Autodesk Inventor part; units mm, degrees
(part 2 of 6)
  arc A582 (128.3559, 101.1967) -> (128.4338, 100.8049) centre (148.5, 105) ccw
  arc A583 (128.7164, 99.628) -> (128.8248, 99.2435) centre (148.5, 105) ccw
  arc A584 (129.1989, 98.0923) -> (129.3371, 97.7175) centre (148.5, 105) ccw
  arc A585 (129.8003, 96.5993) -> (129.9676, 96.2365) centre (148.5, 105) ccw
  arc A586 (130.5171, 95.158) -> (130.7123, 94.8095) centre (148.5, 105) ccw
  arc A587 (131.3447, 93.7774) -> (131.5666, 93.4453) centre (148.5, 105) ccw
  arc A588 (132.2781, 92.466) -> (132.5254, 92.1523) centre (148.5, 105) ccw
  arc A589 (133.3115, 91.2319) -> (133.5827, 90.9386) centre (148.5, 105) ccw
  arc A590 (134.4386, 90.0827) -> (134.7319, 89.8115) centre (148.5, 105) ccw
  arc A591 (135.6523, 89.0254) -> (135.966, 88.7781) centre (148.5, 105) ccw
  arc A592 (136.9453, 88.0666) -> (137.2774, 87.8447) centre (148.5, 105) ccw
  arc A593 (138.3095, 87.2123) -> (138.658, 87.0171) centre (148.5, 105) ccw
  arc A594 (139.7365, 86.4676) -> (140.0993, 86.3003) centre (148.5, 105) ccw
  arc A595 (141.2175, 85.8371) -> (141.5923, 85.6989) centre (148.5, 105) ccw
  arc A596 (142.7435, 85.3248) -> (143.128, 85.2164) centre (148.5, 105) ccw
  arc A597 (144.3049, 84.9338) -> (144.6967, 84.8559) centre (148.5, 105) ccw
  arc A598 (145.8922, 84.6665) -> (146.2889, 84.6196) centre (148.5, 105) ccw
  arc A599 (147.4956, 84.5246) -> (147.8948, 84.5089) centre (148.5, 105) ccw
  arc A600 (149.1052, 84.5089) -> (149.5044, 84.5246) centre (148.5, 105) ccw
  arc A601 (150.7111, 84.6196) -> (151.1078, 84.6665) centre (148.5, 105) ccw
  arc A602 (152.3033, 84.8559) -> (152.6951, 84.9338) centre (148.5, 105) ccw
  arc A603 (153.872, 85.2164) -> (154.2565, 85.3248) centre (148.5, 105) ccw
  arc A604 (155.4077, 85.6989) -> (155.7825, 85.8371) centre (148.5, 105) ccw
  arc A605 (156.9007, 86.3003) -> (157.2635, 86.4676) centre (148.5, 105) ccw
  arc A606 (158.342, 87.0171) -> (158.6905, 87.2123) centre (148.5, 105) ccw
  arc A607 (159.7226, 87.8447) -> (160.0547, 88.0666) centre (148.5, 105) ccw
  arc A608 (161.034, 88.7781) -> (161.3477, 89.0254) centre (148.5, 105) ccw
  arc A609 (162.2681, 89.8115) -> (162.5614, 90.0827) centre (148.5, 105) ccw
  arc A610 (163.4173, 90.9386) -> (163.6885, 91.2319) centre (148.5, 105) ccw
  arc A611 (164.4746, 92.1523) -> (164.7219, 92.466) centre (148.5, 105) ccw
  arc A612 (165.4334, 93.4453) -> (165.6553, 93.7774) centre (148.5, 105) ccw
  arc A613 (166.2877, 94.8095) -> (166.4829, 95.158) centre (148.5, 105) ccw
  arc A614 (167.0324, 96.2365) -> (167.1997, 96.5993) centre (148.5, 105) ccw
  arc A615 (167.6629, 97.7175) -> (167.8011, 98.0923) centre (148.5, 105) ccw
  arc A616 (168.1752, 99.2435) -> (168.2836, 99.628) centre (148.5, 105) ccw
  arc A617 (168.5662, 100.8049) -> (168.6441, 101.1967) centre (148.5, 105) ccw
  arc A618 (168.8335, 102.3922) -> (168.8804, 102.7889) centre (148.5, 105) ccw
  arc A619 (168.9754, 103.9956) -> (168.9911, 104.3948) centre (148.5, 105) ccw
  arc A620 (168.9911, 105.6052) -> (168.9754, 106.0044) centre (148.5, 105) ccw
  arc A621 (168.8804, 107.2111) -> (168.8335, 107.6078) centre (148.5, 105) ccw
  arc A622 (168.6441, 108.8033) -> (168.5662, 109.1951) centre (148.5, 105) ccw
  arc A623 (168.2836, 110.372) -> (168.1752, 110.7565) centre (148.5, 105) ccw
  arc A624 (167.8011, 111.9077) -> (167.6629, 112.2825) centre (148.5, 105) ccw
  arc A625 (167.1997, 113.4007) -> (167.0324, 113.7635) centre (148.5, 105) ccw
  arc A626 (166.4829, 114.842) -> (166.2877, 115.1905) centre (148.5, 105) ccw
  arc A627 (165.6553, 116.2226) -> (165.4334, 116.5547) centre (148.5, 105) ccw
  arc A628 (164.7219, 117.534) -> (164.4746, 117.8477) centre (148.5, 105) ccw
  arc A629 (163.6885, 118.7681) -> (163.4173, 119.0614) centre (148.5, 105) ccw
  arc A630 (162.5614, 119.9173) -> (162.2681, 120.1885) centre (148.5, 105) ccw
  arc A631 (161.3477, 120.9746) -> (161.034, 121.2219) centre (148.5, 105) ccw
  arc A632 (160.0547, 121.9334) -> (159.7226, 122.1553) centre (148.5, 105) ccw
  arc A633 (158.6905, 122.7877) -> (158.342, 122.9829) centre (148.5, 105) ccw
  arc A634 (157.2635, 123.5324) -> (156.9007, 123.6997) centre (148.5, 105) ccw
  arc A635 (155.7825, 124.1629) -> (155.4077, 124.3011) centre (148.5, 105) ccw
  arc A636 (154.2565, 124.6752) -> (153.872, 124.7836) centre (148.5, 105) ccw
  arc A637 (152.6951, 125.0662) -> (152.3033, 125.1441) centre (148.5, 105) ccw
  arc A638 (151.1078, 125.3335) -> (150.7111, 125.3804) centre (148.5, 105) ccw
  arc A639 (149.5044, 125.4754) -> (149.1052, 125.4911) centre (148.5, 105) ccw
  line L0 (126, 105) -> (171, 105)
  line L1 (148.5, 82.5) -> (148.5, 127.5)
  line L2 (189, 125.5) -> (259, 125.5)
  line L3 (189, 117.5) -> (259, 117.5)
  line L4 (189, 109.5) -> (259, 109.5)
  line L5 (189, 101.5) -> (259, 101.5)
  line L6 (189, 93.5) -> (259, 93.5)
  line L7 (189, 85.5) -> (259, 85.5)
  line L8 (189, 77.5) -> (259, 77.5)
  line L9 (189, 69.5) -> (259, 69.5)
  line L10 (189, 61.5) -> (259, 61.5)
  line L11 (189, 53.5) -> (259, 53.5)
  line L12 (189, 45.5) -> (259, 45.5)
  line L13 (189, 37.5) -> (259, 37.5)
  line L14 (189, 29.5) -> (259, 29.5)
  line L15 (189, 125.5) -> (189, 29.5)
  line L16 (259, 125.5) -> (259, 29.5)
  line L17 (224, 117.5) -> (224, 29.5)
  arc A640 (149.1982, 109.7586) -> (149.1615, 109.6213) centre (149.7545, 109.5365) ccw
  arc A641 (149.402, 110.1264) -> (149.1982, 109.7586) centre (150.7515, 109.1382) ccw
  arc A642 (150.0725, 110.7903) -> (149.402, 110.1264) centre (151.8157, 108.3591) ccw
  arc A643 (146.2672, 109.2599) -> (146.3182, 109.1272) centre (146.8478, 109.4071) ccw
  arc A644 (146.2159, 109.6791) -> (146.2672, 109.2599) centre (147.8885, 109.671) ccw
  arc A645 (146.3688, 110.6087) -> (146.2159, 109.6791) centre (149.2074, 109.6645) ccw
  arc A646 (144.1897, 107.1339) -> (144.309, 107.0566) centre (144.5729, 107.5943) ccw
  arc A647 (143.9018, 107.4429) -> (144.1897, 107.1339) centre (145.2598, 108.4195) ccw
  arc A648 (143.4791, 108.2848) -> (143.9018, 107.4429) centre (146.3305, 109.1895) ccw
  arc A649 (143.7586, 104.1928) -> (143.9006, 104.2004) centre (143.7981, 104.7905) ccw
  arc A650 (143.3441, 104.2736) -> (143.7586, 104.1928) centre (143.8687, 105.8619) ccw
  arc A651 (142.5072, 104.7063) -> (143.3441, 104.2736) centre (144.2823, 107.1142) ccw
  arc A652 (145.1386, 101.5601) -> (145.249, 101.6496) centre (144.8192, 102.0668) ccw
  arc A653 (144.7558, 101.3818) -> (145.1386, 101.5601) centre (144.2466, 102.9751) ccw
  arc A654 (143.8244, 101.2399) -> (144.7558, 101.3818) centre (143.8452, 104.2313) ccw
  arc A655 (147.8018, 100.2415) -> (147.8385, 100.3788) centre (147.2456, 100.4636) ccw
  arc A656 (147.5969, 99.8722) -> (147.8018, 100.2415) centre (146.2485, 100.8619) ccw
  arc A657 (146.9268, 99.2099) -> (147.5969, 99.8722) centre (145.1853, 101.6423) ccw
  arc A658 (150.7315, 100.7396) -> (150.6805, 100.8723) centre (150.1509, 100.5924) ccw
  arc A659 (150.7828, 100.3204) -> (150.7315, 100.7396) centre (149.1102, 100.3285) ccw
  arc A660 (150.6299, 99.3908) -> (150.7828, 100.3204) centre (147.7913, 100.335) ccw
  arc A661 (152.8095, 102.8649) -> (152.6903, 102.9423) centre (152.4263, 102.4046) ccw
  arc A662 (153.0974, 102.5559) -> (152.8095, 102.8649) centre (151.7394, 101.5794) ccw
  arc A663 (153.5202, 101.714) -> (153.0974, 102.5559) centre (150.6687, 100.8093) ccw
  arc A664 (153.2414, 105.8058) -> (153.0995, 105.7982) centre (153.202, 105.2081) ccw
  arc A665 (153.656, 105.725) -> (153.2414, 105.8058) centre (153.1314, 104.1367) ccw
  arc A666 (154.4929, 105.2923) -> (153.656, 105.725) centre (152.7177, 102.8844) ccw
  arc A667 (151.8623, 108.4388) -> (151.7519, 108.3493) centre (152.1817, 107.9321) ccw
  arc A668 (152.2451, 108.6171) -> (151.8623, 108.4388) centre (152.7543, 107.0239) ccw
  arc A669 (153.1765, 108.759) -> (152.2451, 108.6171) centre (153.1557, 105.7676) ccw
  arc A670 (147.8392, 109.6213) -> (147.8025, 109.7587) centre (147.2462, 109.5365) ccw
  arc A671 (147.8025, 109.7587) -> (147.5976, 110.128) centre (146.2492, 109.1383) ccw
  arc A672 (147.5976, 110.128) -> (146.9275, 110.7903) centre (145.186, 108.3579) ccw
  arc A673 (145.2491, 108.3503) -> (145.1386, 108.4399) centre (144.8192, 107.9332) ccw
  arc A674 (145.1386, 108.4399) -> (144.7558, 108.6182) centre (144.2466, 107.0249) ccw
  arc A675 (144.7558, 108.6182) -> (143.8244, 108.7601) centre (143.8452, 105.7687) ccw
  arc A676 (143.9007, 105.7996) -> (143.7586, 105.8072) centre (143.7981, 105.2095) ccw
  arc A677 (143.7586, 105.8072) -> (143.3441, 105.7264) centre (143.8687, 104.1381) ccw
  arc A678 (143.3441, 105.7264) -> (142.5072, 105.2937) centre (144.2823, 102.8858) ccw
  arc A679 (144.309, 102.9435) -> (144.1897, 102.8661) centre (144.5729, 102.4057) ccw
  arc A680 (144.1897, 102.8661) -> (143.9018, 102.5571) centre (145.2598, 101.5805) ccw
  arc A681 (143.9018, 102.5571) -> (143.4791, 101.7152) centre (146.3305, 100.8105) ccw
  arc A682 (146.3189, 100.8726) -> (146.2679, 100.7399) centre (146.8485, 100.5927) ccw
  arc A683 (146.2679, 100.7399) -> (146.2166, 100.3207) centre (147.8892, 100.3288) ccw
  arc A684 (146.2166, 100.3207) -> (146.3695, 99.391) centre (149.2081, 100.3352) ccw
  arc A685 (149.1608, 100.3787) -> (149.1975, 100.2413) centre (149.7538, 100.4635) ccw
  arc A686 (149.1975, 100.2413) -> (149.4024, 99.872) centre (150.7508, 100.8617) ccw
  arc A687 (149.4024, 99.872) -> (150.0725, 99.2097) centre (151.814, 101.6421) ccw
  arc A688 (151.7509, 101.6497) -> (151.8614, 101.5601) centre (152.1808, 102.0668) ccw
  arc A689 (151.8614, 101.5601) -> (152.2442, 101.3818) centre (152.7534, 102.9751) ccw
  arc A690 (152.2442, 101.3818) -> (153.1756, 101.2399) centre (153.1548, 104.2313) ccw
  arc A691 (153.0993, 104.2004) -> (153.2414, 104.1928) centre (153.2019, 104.7905) ccw
  arc A692 (153.2414, 104.1928) -> (153.6559, 104.2736) centre (153.1313, 105.8619) ccw
  arc A693 (153.6559, 104.2736) -> (154.4928, 104.7063) centre (152.7177, 107.1142) ccw
  arc A694 (152.691, 107.0565) -> (152.8103, 107.1339) centre (152.4271, 107.5943) ccw
  arc A695 (152.8103, 107.1339) -> (153.0982, 107.4429) centre (151.7402, 108.4195) ccw
  arc A696 (153.0982, 107.4429) -> (153.5209, 108.2848) centre (150.6695, 109.1895) ccw
  arc A697 (150.6818, 109.1272) -> (150.7328, 109.2599) centre (150.1522, 109.4071) ccw
  arc A698 (150.7328, 109.2599) -> (150.7841, 109.6791) centre (149.1115, 109.671) ccw
  arc A699 (150.7841, 109.6791) -> (150.6312, 110.6087) centre (147.7926, 109.6645) ccw
  arc A700 (149.0314, 108.7125) -> (147.9691, 108.7126) centre (148.5, 105) ccw
  arc A701 (146.7471, 108.3155) -> (145.8883, 107.6915) centre (148.5, 105) ccw
  arc A702 (145.1331, 106.652) -> (144.8051, 105.6424) centre (148.5, 105) ccw
  arc A703 (144.8051, 104.3575) -> (145.1332, 103.3479) centre (148.5, 105) ccw
  arc A704 (145.8884, 102.3084) -> (146.7478, 101.6841) centre (148.5, 105) ccw
  arc A705 (147.9686, 101.2875) -> (149.0308, 101.2874) centre (148.5, 105) ccw
  arc A706 (150.2516, 101.6838) -> (151.1117, 102.3085) centre (148.5, 105) ccw
  arc A707 (151.8663, 103.3467) -> (152.1949, 104.3576) centre (148.5, 105) ccw
  arc A708 (152.1951, 105.6411) -> (151.8668, 106.6521) centre (148.5, 105) ccw
  arc A709 (151.1126, 107.6906) -> (150.2528, 108.3155) centre (148.5, 105) ccw
  arc A710 (146.9275, 110.7903) -> (146.3688, 110.6087) centre (148.5, 105) ccw
  arc A711 (143.8244, 108.7601) -> (143.4791, 108.2848) centre (148.5, 105) ccw
  arc A712 (142.5072, 105.2937) -> (142.5072, 104.7063) centre (148.5, 105) ccw
  arc A713 (143.4791, 101.7152) -> (143.8244, 101.2399) centre (148.5, 105) ccw
  arc A714 (146.3695, 99.391) -> (146.9268, 99.2099) centre (148.5, 105) ccw
  arc A715 (150.0725, 99.2097) -> (150.6299, 99.3908) centre (148.5, 105) ccw
  arc A716 (153.1756, 101.2399) -> (153.5202, 101.714) centre (148.5, 105) ccw
  arc A717 (154.4928, 104.7063) -> (154.4929, 105.2923) centre (148.5, 105) ccw
  arc A718 (153.5209, 108.2848) -> (153.1765, 108.759) centre (148.5, 105) ccw
  arc A719 (150.6312, 110.6087) -> (150.0725, 110.7903) centre (148.5, 105) ccw
  line L18 (149.0314, 108.7125) -> (149.1615, 109.6213)
  line L19 (146.7471, 108.3155) -> (146.3182, 109.1272)
  line L20 (145.1331, 106.652) -> (144.309, 107.0566)
  line L21 (144.8051, 104.3575) -> (143.9006, 104.2004)
  line L22 (145.8884, 102.3084) -> (145.249, 101.6496)
  line L23 (147.9686, 101.2875) -> (147.8385, 100.3788)
  line L24 (150.2516, 101.6838) -> (150.6805, 100.8723)
  line L25 (151.8663, 103.3467) -> (152.6903, 102.9423)
  line L26 (152.1951, 105.6411) -> (153.0995, 105.7982)
  line L27 (151.1126, 107.6906) -> (151.7519, 108.3493)
  line L28 (147.9691, 108.7126) -> (147.8392, 109.6213)
  line L29 (145.8883, 107.6915) -> (145.2491, 108.3503)
  line L30 (144.8051, 105.6424) -> (143.9007, 105.7996)
  line L31 (145.1332, 103.3479) -> (144.309, 102.9435)
  line L32 (146.7478, 101.6841) -> (146.3189, 100.8726)
  line L33 (149.0308, 101.2874) -> (149.1608, 100.3787)
  line L34 (151.1117, 102.3085) -> (151.7509, 101.6497)
  line L35 (152.1949, 104.3576) -> (153.0993, 104.2004)
  line L36 (151.8668, 106.6521) -> (152.691, 107.0565)
  line L37 (150.2528, 108.3155) -> (150.6818, 109.1272)
  line L38 (140.5, 105) -> (156.5, 105)
  line L39 (148.5, 97) -> (148.5, 113)
  line L40 (174.5, 111) -> (244.5, 111)
  line L41 (174.5, 103) -> (244.5, 103)
  line L42 (174.5, 95) -> (244.5, 95)
  line L43 (174.5, 87) -> (244.5, 87)
  line L44 (174.5, 79) -> (244.5, 79)
  line L45 (174.5, 71) -> (244.5, 71)
  line L46 (174.5, 63) -> (244.5, 63)
  line L47 (174.5, 55) -> (244.5, 55)
  line L48 (174.5, 47) -> (244.5, 47)
  line L49 (174.5, 39) -> (244.5, 39)
  line L50 (174.5, 31) -> (244.5, 31)
  line L51 (174.5, 23) -> (244.5, 23)
  line L52 (174.5, 15) -> (244.5, 15)
  line L53 (174.5, 111) -> (174.5, 15)
  line L54 (244.5, 111) -> (244.5, 15)
  line L55 (209.5, 103) -> (209.5, 15)
  point P0 (0, 0)
  point P1 (195, 119.5)
  point P2 (197.5, 111.5)
  point P3 (197.5, 103.5)
  point P4 (195, 95.5)
  point P5 (197.5, 87.5)
  point P6 (192.5, 79.5)
  point P7 (195, 71.5)
  point P8 (195, 63.5)
  point P9 (195, 55.5)
  point P10 (197.5, 47.5)
  point P11 (197.5, 39.5)
  point P12 (195, 31.5)
  point P13 (225, 111.5)
  point P14 (240, 103.5)
  point P15 (238.75, 95.5)
  point P16 (237.5, 87.5)
  point P17 (240, 79.5)
  point P18 (233.75, 71.5)
  point P19 (240, 63.5)
  point P20 (236.25, 55.5)
  point P21 (235, 47.5)
  point P22 (242.5, 39.5)
  point P23 (242.5, 31.5)
  point P24 (149.5, 141)
  point P25 (149.5, 135)
  point P26 (165.6875, 141)
  point P27 (167.8125, 135)
  point P28 (180.5, 105)
  point P29 (183, 97)
  point P30 (183, 89)
  point P31 (180.5, 81)
  point P32 (183, 73)
  point P33 (178, 65)
  point P34 (180.5, 57)
  point P35 (180.5, 49)
  point P36 (180.5, 41)
  point P37 (183, 33)
  point P38 (183, 25)
  point P39 (180.5, 17)
  point P40 (210.5, 97)
  point P41 (225.5, 89)
  point P42 (226.75, 81)
  point P43 (223, 73)
  point P44 (225.5, 65)
  point P45 (220.5, 57)
  point P46 (225.5, 49)
  point P47 (224.25, 41)
  point P48 (220.5, 33)
  point P49 (228, 25)
  point P50 (228, 17)
  point P51 (149.5, 126.5)
  point P52 (149.5, 120.5)
  point P53 (167.8125, 126.5)
  point P54 (168.875, 120.5)
  constraints: 1120 point on circle, 560 centre point, 534 equal radius, 410 tangent, 104 end point, 84 horizontal, 26 parallel, 9 concentric, 4 midpoint, 4 perpendicular, 2 horizontal alignment, 2 vertical alignment, 586 other
extrude "押し出し1" add sketch "スケッチ1" along normal blind 3 contours A1 A2 A639 A479 A478 A477 A559 A237 A238 A239 A638 A476 A475 A474 A558 A234 A235 A236 A637 A473 A472 A471 A557 A231 A232 A233 A636 A470 A469 A468 A556 A228 A229 A230 A635 A467 A466 A465 A555 A225 A226 A227 A634 A464 A463 A462 A554 A222 A223 A224 A633 A461 A460 A459 A553 A219 A220 A221 A632 A458 A457 A456 A552 A216 A217 A218 A631 A455 A454 A453 A551 A213 A214 A215 A630 A452 A451 A450 A550 A210 A211 A212 A629 A449 A448 A447 A549 A207 A208 A209 A628 A446 A445 A444 A548 A204 A205 A206 A627 A443 A442 A441 A547 A201 A202 A203 A626 A440 A439 A438 A546 A198 A199 A200 A625 A437 A436 A435 A545 A195 A196 A197 A624 A434 A433 A432 A544 A192 A193 A194 A623 A431 A430 A429 A543 A189 A190 A191 A622 A428 A427 A426 A542 A186 A187 A188 A621 A425 A424 A423 A541 A183 A184 A185 A620 A422 A421 A420 A540 L0 A717 A666 A665 A664 L26 A708 L36 A694 A695 A696 A718 A669 A668 A667 L27 A709 L37 A697 A698 A699 A719 A642 A641 A640 L18 A700 L1 A480 A0 | L1 A700 L28 A670 A671 A672 A710 A645 A644 A643 L19 A701 L29 A673 A674 A675 A711 A648 A647 A646 L20 A702 L30 A676 A677 A678 A712 L0 A500 A60 A61 A62 A579 A299 A298 A297 A499 A57 A58 A59 A578 A296 A295 A294 A498 A54 A55 A56 A577 A293 A292 A291 A497 A51 A52 A53 A576 A290 A289 A288 A496 A48 A49 A50 A575 A287 A286 A285 A495 A45 A46 A47 A574 A284 A283 A282 A494 A42 A43 A44 A573 A281 A280 A279 A493 A39 A40 A41 A572 A278 A277 A276 A492 A36 A37 A38 A571 A275 A274 A273 A491 A33 A34 A35 A570 A272 A271 A270 A490 A30 A31 A32 A569 A269 A268 A267 A489 A27 A28 A29 A568 A266 A265 A264 A488 A24 A25 A26 A567 A263 A262 A261 A487 A21 A22 A23 A566 A260 A259 A258 A486 A18 A19 A20 A565 A257 A256 A255 A485 A15 A16 A17 A564 A254 A253 A252 A484 A12 A13 A14 A563 A251 A250 A249 A483 A9 A10 A11 A562 A248 A247 A246 A482 A6 A7 A8 A561 A245 A244 A243 A481 A3 A4 A5 A560 A242 A241 A240 A480 | A700 L18 A640 A641 A642 A719 A699 A698 A697 L37 A709 L27 A667 A668 A669 A718 A696 A695 A694 L36 A708 L26 A664 A665 A666 A717 L0 L1 | L1 L0 A712 A678 A677 A676 L30 A702 L20 A646 A647 A648 A711 A675 A674 A673 L29 A701 L19 A643 A644 A645 A710 A672 A671 A670 L28 A700 | L1 A705 L23 A655 A656 A657 A714 A684 A683 A682 L32 A704 L22 A652 A653 A654 A713 A681 A680 A679 L31 A703 L21 A649 A650 A651 A712 L0 | L0 A717 A693 A692 A691 L35 A707 L25 A661 A662 A663 A716 A690 A689 A688 L34 A706 L24 A658 A659 A660 A715 A687 A686 A685 L33 A705 L1 | A712 A651 A650 A649 L21 A703 L31 A679 A680 A681 A713 A654 A653 A652 L22 A704 L32 A682 A683 A684 A714 A657 A656 A655 L23 A705 L1 A520 A120 A121 A122 A599 A359 A358 A357 A519 A117 A118 A119 A598 A356 A355 A354 A518 A114 A115 A116 A597 A353 A352 A351 A517 A111 A112 A113 A596 A350 A349 A348 A516 A108 A109 A110 A595 A347 A346 A345 A515 A105 A106 A107 A594 A344 A343 A342 A514 A102 A103 A104 A593 A341 A340 A339 A513 A99 A100 A101 A592 A338 A337 A336 A512 A96 A97 A98 A591 A335 A334 A333 A511 A93 A94 A95 A590 A332 A331 A330 A510 A90 A91 A92 A589 A329 A328 A327 A509 A87 A88 A89 A588 A326 A325 A324 A508 A84 A85 A86 A587 A323 A322 A321 A507 A81 A82 A83 A586 A320 A319 A318 A506 A78 A79 A80 A585 A317 A316 A315 A505 A75 A76 A77 A584 A314 A313 A312 A504 A72 A73 A74 A583 A311 A310 A309 A503 A69 A70 A71 A582 A308 A307 A306 A502 A66 A67 A68 A581 A305 A304 A303 A501 A63 A64 A65 A580 A302 A301 A300 A500 L0 | L0 A540 A180 A181 A182 A619 A419 A418 A417 A539 A177 A178 A179 A618 A416 A415 A414 A538 A174 A175 A176 A617 A413 A412 A411 A537 A171 A172 A173 A616 A410 A409 A408 A536 A168 A169 A170 A615 A407 A406 A405 A535 A165 A166 A167 A614 A404 A403 A402 A534 A162 A163 A164 A613 A401 A400 A399 A533 A159 A160 A161 A612 A398 A397 A396 A532 A156 A157 A158 A611 A395 A394 A393 A531 A153 A154 A155 A610 A392 A391 A390 A530 A150 A151 A152 A609 A389 A388 A387 A529 A147 A148 A149 A608 A386 A385 A384 A528 A144 A145 A146 A607 A383 A382 A381 A527 A141 A142 A143 A606 A380 A379 A378 A526 A138 A139 A140 A605 A377 A376 A375 A525 A135 A136 A137 A604 A374 A373 A372 A524 A132 A133 A134 A603 A371 A370 A369 A523 A129 A130 A131 A602 A368 A367 A366 A522 A126 A127 A128 A601 A365 A364 A363 A521 A123 A124 A125 A600 A362 A361 A360 A520 L1 A705 L33 A685 A686 A687 A715 A660 A659 A658 L24 A706 L34 A688 A689 A690 A716 A663 A662 A661 L25 A707 L35 A691 A692 A693 A717
extrude "押し出し2" add sketch "スケッチ1" against normal blind 5 contours A700 L18 A640 A641 A642 A719 A699 A698 A697 L37 A709 L27 A667 A668 A669 A718 A696 A695 A694 L36 A708 L26 A664 A665 A666 A717 L0 L1 | L1 L0 A712 A678 A677 A676 L30 A702 L20 A646 A647 A648 A711 A675 A674 A673 L29 A701 L19 A643 A644 A645 A710 A672 A671 A670 L28 A700 | L1 A705 L23 A655 A656 A657 A714 A684 A683 A682 L32 A704 L22 A652 A653 A654 A713 A681 A680 A679 L31 A703 L21 A649 A650 A651 A712 L0 | L0 A717 A693 A692 A691 L35 A707 L25 A661 A662 A663 A716 A690 A689 A688 L34 A706 L24 A658 A659 A660 A715 A687 A686 A685 L33 A705 L1
sketch "スケッチ2" plane through (0, 0, -5) normal (0, 0, -1) x (-1, 0, 0)
  line L0 (-149.1615, 109.6213) -> (-149.0314, 108.7125) projected
  arc A0 (-147.9691, 108.7126) -> (-149.0314, 108.7125) centre (-148.5, 105) ccw projected
  line L1 (-147.9691, 108.7126) -> (-147.8392, 109.6213) projected
  arc A1 (-147.8025, 109.7587) -> (-147.8392, 109.6213) centre (-147.2462, 109.5365) ccw projected
  arc A2 (-147.5976, 110.128) -> (-147.8025, 109.7587) centre (-146.2492, 109.1383) ccw projected
  arc A3 (-146.9275, 110.7903) -> (-147.5976, 110.128) centre (-145.186, 108.3579) ccw projected
  arc A4 (-146.3688, 110.6087) -> (-146.9275, 110.7903) centre (-148.5, 105) ccw projected
  arc A5 (-146.2159, 109.6791) -> (-146.3688, 110.6087) centre (-149.2074, 109.6645) ccw projected
  arc A6 (-146.2672, 109.2599) -> (-146.2159, 109.6791) centre (-147.8885, 109.671) ccw projected
  arc A7 (-146.3182, 109.1272) -> (-146.2672, 109.2599) centre (-146.8478, 109.4071) ccw projected
  line L2 (-146.3182, 109.1272) -> (-146.7471, 108.3155) projected
  arc A8 (-145.8883, 107.6915) -> (-146.7471, 108.3155) centre (-148.5, 105) ccw projected
  line L3 (-145.8883, 107.6915) -> (-145.2491, 108.3503) projected
  arc A9 (-145.1386, 108.4399) -> (-145.2491, 108.3503) centre (-144.8192, 107.9332) ccw projected
  arc A10 (-144.7558, 108.6182) -> (-145.1386, 108.4399) centre (-144.2466, 107.0249) ccw projected
  arc A11 (-143.8244, 108.7601) -> (-144.7558, 108.6182) centre (-143.8452, 105.7687) ccw projected
  arc A12 (-143.4791, 108.2848) -> (-143.8244, 108.7601) centre (-148.5, 105) ccw projected
  arc A13 (-143.9018, 107.4429) -> (-143.4791, 108.2848) centre (-146.3305, 109.1895) ccw projected
  arc A14 (-144.1897, 107.1339) -> (-143.9018, 107.4429) centre (-145.2598, 108.4195) ccw projected
  arc A15 (-144.309, 107.0566) -> (-144.1897, 107.1339) centre (-144.5729, 107.5943) ccw projected
  line L4 (-144.309, 107.0566) -> (-145.1331, 106.652) projected
  arc A16 (-144.8051, 105.6424) -> (-145.1331, 106.652) centre (-148.5, 105) ccw projected
  line L5 (-144.8051, 105.6424) -> (-143.9007, 105.7996) projected
  arc A17 (-143.7586, 105.8072) -> (-143.9007, 105.7996) centre (-143.7981, 105.2095) ccw projected
  arc A18 (-143.3441, 105.7264) -> (-143.7586, 105.8072) centre (-143.8687, 104.1381) ccw projected
  arc A19 (-142.5072, 105.2937) -> (-143.3441, 105.7264) centre (-144.2823, 102.8858) ccw projected
  arc A20 (-142.5072, 104.7063) -> (-142.5072, 105.2937) centre (-148.5, 105) ccw projected
  arc A21 (-143.3441, 104.2736) -> (-142.5072, 104.7063) centre (-144.2823, 107.1142) ccw projected
  arc A22 (-143.7586, 104.1928) -> (-143.3441, 104.2736) centre (-143.8687, 105.8619) ccw projected
  arc A23 (-143.9006, 104.2004) -> (-143.7586, 104.1928) centre (-143.7981, 104.7905) ccw projected
  line L6 (-143.9006, 104.2004) -> (-144.8051, 104.3575) projected
  arc A24 (-145.1332, 103.3479) -> (-144.8051, 104.3575) centre (-148.5, 105) ccw projected
  line L7 (-145.1332, 103.3479) -> (-144.309, 102.9435) projected
  arc A25 (-144.1897, 102.8661) -> (-144.309, 102.9435) centre (-144.5729, 102.4057) ccw projected
  arc A26 (-143.9018, 102.5571) -> (-144.1897, 102.8661) centre (-145.2598, 101.5805) ccw projected
  arc A27 (-143.4791, 101.7152) -> (-143.9018, 102.5571) centre (-146.3305, 100.8105) ccw projected
  arc A28 (-143.8244, 101.2399) -> (-143.4791, 101.7152) centre (-148.5, 105) ccw projected
  arc A29 (-144.7558, 101.3818) -> (-143.8244, 101.2399) centre (-143.8452, 104.2313) ccw projected
  arc A30 (-145.1386, 101.5601) -> (-144.7558, 101.3818) centre (-144.2466, 102.9751) ccw projected
  arc A31 (-145.249, 101.6496) -> (-145.1386, 101.5601) centre (-144.8192, 102.0668) ccw projected
  line L8 (-145.249, 101.6496) -> (-145.8884, 102.3084) projected
  arc A32 (-146.7478, 101.6841) -> (-145.8884, 102.3084) centre (-148.5, 105) ccw projected
  line L9 (-146.7478, 101.6841) -> (-146.3189, 100.8726) projected
  arc A33 (-146.2679, 100.7399) -> (-146.3189, 100.8726) centre (-146.8485, 100.5927) ccw projected
  arc A34 (-146.2166, 100.3207) -> (-146.2679, 100.7399) centre (-147.8892, 100.3288) ccw projected
  arc A35 (-146.3695, 99.391) -> (-146.2166, 100.3207) centre (-149.2081, 100.3352) ccw projected
  arc A36 (-146.9268, 99.2099) -> (-146.3695, 99.391) centre (-148.5, 105) ccw projected
  arc A37 (-147.5969, 99.8722) -> (-146.9268, 99.2099) centre (-145.1853, 101.6423) ccw projected
  arc A38 (-147.8018, 100.2415) -> (-147.5969, 99.8722) centre (-146.2485, 100.8619) ccw projected
  arc A39 (-147.8385, 100.3788) -> (-147.8018, 100.2415) centre (-147.2456, 100.4636) ccw projected
  line L10 (-147.8385, 100.3788) -> (-147.9686, 101.2875) projected
  arc A40 (-149.0308, 101.2874) -> (-147.9686, 101.2875) centre (-148.5, 105) ccw projected
  line L11 (-149.0308, 101.2874) -> (-149.1608, 100.3787) projected
  arc A41 (-149.1975, 100.2413) -> (-149.1608, 100.3787) centre (-149.7538, 100.4635) ccw projected
  arc A42 (-149.4024, 99.872) -> (-149.1975, 100.2413) centre (-150.7508, 100.8617) ccw projected
  arc A43 (-150.0725, 99.2097) -> (-149.4024, 99.872) centre (-151.814, 101.6421) ccw projected
  arc A44 (-150.6299, 99.3908) -> (-150.0725, 99.2097) centre (-148.5, 105) ccw projected
  arc A45 (-150.7828, 100.3204) -> (-150.6299, 99.3908) centre (-147.7913, 100.335) ccw projected
  arc A46 (-150.7315, 100.7396) -> (-150.7828, 100.3204) centre (-149.1102, 100.3285) ccw projected
  arc A47 (-150.6805, 100.8723) -> (-150.7315, 100.7396) centre (-150.1509, 100.5924) ccw projected
  line L12 (-150.6805, 100.8723) -> (-150.2516, 101.6838) projected
  arc A48 (-151.1117, 102.3085) -> (-150.2516, 101.6838) centre (-148.5, 105) ccw projected
  line L13 (-151.1117, 102.3085) -> (-151.7509, 101.6497) projected
  arc A49 (-151.8614, 101.5601) -> (-151.7509, 101.6497) centre (-152.1808, 102.0668) ccw projected
  arc A50 (-152.2442, 101.3818) -> (-151.8614, 101.5601) centre (-152.7534, 102.9751) ccw projected
  arc A51 (-153.1756, 101.2399) -> (-152.2442, 101.3818) centre (-153.1548, 104.2313) ccw projected
  arc A52 (-153.5202, 101.714) -> (-153.1756, 101.2399) centre (-148.5, 105) ccw projected
  arc A53 (-153.0974, 102.5559) -> (-153.5202, 101.714) centre (-150.6687, 100.8093) ccw projected
  arc A54 (-152.8095, 102.8649) -> (-153.0974, 102.5559) centre (-151.7394, 101.5794) ccw projected
  arc A55 (-152.6903, 102.9423) -> (-152.8095, 102.8649) centre (-152.4263, 102.4046) ccw projected
  line L14 (-152.6903, 102.9423) -> (-151.8663, 103.3467) projected
  arc A56 (-152.1949, 104.3576) -> (-151.8663, 103.3467) centre (-148.5, 105) ccw projected
  line L15 (-152.1949, 104.3576) -> (-153.0993, 104.2004) projected
  arc A57 (-153.2414, 104.1928) -> (-153.0993, 104.2004) centre (-153.2019, 104.7905) ccw projected
  arc A58 (-153.6559, 104.2736) -> (-153.2414, 104.1928) centre (-153.1313, 105.8619) ccw projected
  arc A59 (-154.4928, 104.7063) -> (-153.6559, 104.2736) centre (-152.7177, 107.1142) ccw projected
  arc A60 (-154.4929, 105.2923) -> (-154.4928, 104.7063) centre (-148.5, 105) ccw projected
  arc A61 (-153.656, 105.725) -> (-154.4929, 105.2923) centre (-152.7177, 102.8844) ccw projected
  arc A62 (-153.2414, 105.8058) -> (-153.656, 105.725) centre (-153.1314, 104.1367) ccw projected
  arc A63 (-153.0995, 105.7982) -> (-153.2414, 105.8058) centre (-153.202, 105.2081) ccw projected
  line L16 (-153.0995, 105.7982) -> (-152.1951, 105.6411) projected
  arc A64 (-151.8668, 106.6521) -> (-152.1951, 105.6411) centre (-148.5, 105) ccw projected
  line L17 (-151.8668, 106.6521) -> (-152.691, 107.0565) projected
  arc A65 (-152.8103, 107.1339) -> (-152.691, 107.0565) centre (-152.4271, 107.5943) ccw projected
  arc A66 (-153.0982, 107.4429) -> (-152.8103, 107.1339) centre (-151.7402, 108.4195) ccw projected
  arc A67 (-153.5209, 108.2848) -> (-153.0982, 107.4429) centre (-150.6695, 109.1895) ccw projected
  arc A68 (-153.1765, 108.759) -> (-153.5209, 108.2848) centre (-148.5, 105) ccw projected
  arc A69 (-152.2451, 108.6171) -> (-153.1765, 108.759) centre (-153.1557, 105.7676) ccw projected
  arc A70 (-151.8623, 108.4388) -> (-152.2451, 108.6171) centre (-152.7543, 107.0239) ccw projected
  arc A71 (-151.7519, 108.3493) -> (-151.8623, 108.4388) centre (-152.1817, 107.9321) ccw projected
  line L18 (-151.7519, 108.3493) -> (-151.1126, 107.6906) projected
  arc A72 (-150.2528, 108.3155) -> (-151.1126, 107.6906) centre (-148.5, 105) ccw projected
  line L19 (-150.2528, 108.3155) -> (-150.6818, 109.1272) projected
  arc A73 (-150.7328, 109.2599) -> (-150.6818, 109.1272) centre (-150.1522, 109.4071) ccw projected
  arc A74 (-150.7841, 109.6791) -> (-150.7328, 109.2599) centre (-149.1115, 109.671) ccw projected
  arc A75 (-150.6312, 110.6087) -> (-150.7841, 109.6791) centre (-147.7926, 109.6645) ccw projected
  arc A76 (-150.0725, 110.7903) -> (-150.6312, 110.6087) centre (-148.5, 105) ccw projected
  arc A77 (-149.402, 110.1264) -> (-150.0725, 110.7903) centre (-151.8157, 108.3591) ccw projected
  arc A78 (-149.1982, 109.7586) -> (-149.402, 110.1264) centre (-150.7515, 109.1382) ccw projected
  arc A79 (-149.1615, 109.6213) -> (-149.1982, 109.7586) centre (-149.7545, 109.5365) ccw projected
  point P0 (0, 0)
hole "穴1" at (148.5, 105, -5) direction (0, 0, 1) diameter 4 end through all
sketch "スケッチ3" plane through (0, 0, 0) normal (0, 0, -1) x (-1, 0, 0)
  circle A0 centre (-148.5, 105) radius 2 projected
  line L0 (-149.1615, 109.6213) -> (-149.0314, 108.7125) projected
  arc A1 (-147.9691, 108.7126) -> (-149.0314, 108.7125) centre (-148.5, 105) ccw projected
  line L1 (-147.9691, 108.7126) -> (-147.8392, 109.6213) projected
  arc A2 (-147.8025, 109.7587) -> (-147.8392, 109.6213) centre (-147.2462, 109.5365) ccw projected
  arc A3 (-147.5976, 110.128) -> (-147.8025, 109.7587) centre (-146.2492, 109.1383) ccw projected
  arc A4 (-146.9275, 110.7903) -> (-147.5976, 110.128) centre (-145.186, 108.3579) ccw projected
  arc A5 (-146.3688, 110.6087) -> (-146.9275, 110.7903) centre (-148.5, 105) ccw projected
  arc A6 (-146.2159, 109.6791) -> (-146.3688, 110.6087) centre (-149.2074, 109.6645) ccw projected
  arc A7 (-146.2672, 109.2599) -> (-146.2159, 109.6791) centre (-147.8885, 109.671) ccw projected
  arc A8 (-146.3182, 109.1272) -> (-146.2672, 109.2599) centre (-146.8478, 109.4071) ccw projected
  line L2 (-146.3182, 109.1272) -> (-146.7471, 108.3155) projected
  arc A9 (-145.8883, 107.6915) -> (-146.7471, 108.3155) centre (-148.5, 105) ccw projected
  line L3 (-145.8883, 107.6915) -> (-145.2491, 108.3503) projected
  arc A10 (-145.1386, 108.4399) -> (-145.2491, 108.3503) centre (-144.8192, 107.9332) ccw projected
  arc A11 (-144.7558, 108.6182) -> (-145.1386, 108.4399) centre (-144.2466, 107.0249) ccw projected
  arc A12 (-143.8244, 108.7601) -> (-144.7558, 108.6182) centre (-143.8452, 105.7687) ccw projected
  arc A13 (-143.4791, 108.2848) -> (-143.8244, 108.7601) centre (-148.5, 105) ccw projected
  arc A14 (-143.9018, 107.4429) -> (-143.4791, 108.2848) centre (-146.3305, 109.1895) ccw projected
  arc A15 (-144.1897, 107.1339) -> (-143.9018, 107.4429) centre (-145.2598, 108.4195) ccw projected
  arc A16 (-144.309, 107.0566) -> (-144.1897, 107.1339) centre (-144.5729, 107.5943) ccw projected
  line L4 (-144.309, 107.0566) -> (-145.1331, 106.652) projected
  arc A17 (-144.8051, 105.6424) -> (-145.1331, 106.652) centre (-148.5, 105) ccw projected
  line L5 (-144.8051, 105.6424) -> (-143.9007, 105.7996) projected
  arc A18 (-143.7586, 105.8072) -> (-143.9007, 105.7996) centre (-143.7981, 105.2095) ccw projected
  arc A19 (-143.3441, 105.7264) -> (-143.7586, 105.8072) centre (-143.8687, 104.1381) ccw projected
  arc A20 (-142.5072, 105.2937) -> (-143.3441, 105.7264) centre (-144.2823, 102.8858) ccw projected
  arc A21 (-142.5072, 104.7063) -> (-142.5072, 105.2937) centre (-148.5, 105) ccw projected
  arc A22 (-143.3441, 104.2736) -> (-142.5072, 104.7063) centre (-144.2823, 107.1142) ccw projected
  arc A23 (-143.7586, 104.1928) -> (-143.3441, 104.2736) centre (-143.8687, 105.8619) ccw projected
  arc A24 (-143.9006, 104.2004) -> (-143.7586, 104.1928) centre (-143.7981, 104.7905) ccw projected
  line L6 (-143.9006, 104.2004) -> (-144.8051, 104.3575) projected
  arc A25 (-145.1332, 103.3479) -> (-144.8051, 104.3575) centre (-148.5, 105) ccw projected
  line L7 (-145.1332, 103.3479) -> (-144.309, 102.9435) projected
  arc A26 (-144.1897, 102.8661) -> (-144.309, 102.9435) centre (-144.5729, 102.4057) ccw projected
  arc A27 (-143.9018, 102.5571) -> (-144.1897, 102.8661) centre (-145.2598, 101.5805) ccw projected
  arc A28 (-143.4791, 101.7152) -> (-143.9018, 102.5571) centre (-146.3305, 100.8105) ccw projected
  arc A29 (-143.8244, 101.2399) -> (-143.4791, 101.7152) centre (-148.5, 105) ccw projected
  arc A30 (-144.7558, 101.3818) -> (-143.8244, 101.2399) centre (-143.8452, 104.2313) ccw projected
  arc A31 (-145.1386, 101.5601) -> (-144.7558, 101.3818) centre (-144.2466, 102.9751) ccw projected
  arc A32 (-145.249, 101.6496) -> (-145.1386, 101.5601) centre (-144.8192, 102.0668) ccw projected
  line L8 (-145.249, 101.6496) -> (-145.8884, 102.3084) projected
  arc A33 (-146.7478, 101.6841) -> (-145.8884, 102.3084) centre (-148.5, 105) ccw projected
  line L9 (-146.7478, 101.6841) -> (-146.3189, 100.8726) projected
  arc A34 (-146.2679, 100.7399) -> (-146.3189, 100.8726) centre (-146.8485, 100.5927) ccw projected
  arc A35 (-146.2166, 100.3207) -> (-146.2679, 100.7399) centre (-147.8892, 100.3288) ccw projected
  arc A36 (-146.3695, 99.391) -> (-146.2166, 100.3207) centre (-149.2081, 100.3352) ccw projected
  arc A37 (-146.9268, 99.2099) -> (-146.3695, 99.391) centre (-148.5, 105) ccw projected
  arc A38 (-147.5969, 99.8722) -> (-146.9268, 99.2099) centre (-145.1853, 101.6423) ccw projected
  arc A39 (-147.8018, 100.2415) -> (-147.5969, 99.8722) centre (-146.2485, 100.8619) ccw projected
  arc A40 (-147.8385, 100.3788) -> (-147.8018, 100.2415) centre (-147.2456, 100.4636) ccw projected
  line L10 (-147.8385, 100.3788) -> (-147.9686, 101.2875) projected
  arc A41 (-149.0308, 101.2874) -> (-147.9686, 101.2875) centre (-148.5, 105) ccw projected
  line L11 (-149.0308, 101.2874) -> (-149.1608, 100.3787) projected
  arc A42 (-149.1975, 100.2413) -> (-149.1608, 100.3787) centre (-149.7538, 100.4635) ccw projected
  arc A43 (-149.4024, 99.872) -> (-149.1975, 100.2413) centre (-150.7508, 100.8617) ccw projected
  arc A44 (-150.0725, 99.2097) -> (-149.4024, 99.872) centre (-151.814, 101.6421) ccw projected
  arc A45 (-150.6299, 99.3908) -> (-150.0725, 99.2097) centre (-148.5, 105) ccw projected
  arc A46 (-150.7828, 100.3204) -> (-150.6299, 99.3908) centre (-147.7913, 100.335) ccw projected
  arc A47 (-150.7315, 100.7396) -> (-150.7828, 100.3204) centre (-149.1102, 100.3285) ccw projected
  arc A48 (-150.6805, 100.8723) -> (-150.7315, 100.7396) centre (-150.1509, 100.5924) ccw projected
  line L12 (-150.6805, 100.8723) -> (-150.2516, 101.6838) projected
  arc A49 (-151.1117, 102.3085) -> (-150.2516, 101.6838) centre (-148.5, 105) ccw projected
  line L13 (-151.1117, 102.3085) -> (-151.7509, 101.6497) projected
  arc A50 (-151.8614, 101.5601) -> (-151.7509, 101.6497) centre (-152.1808, 102.0668) ccw projected
  arc A51 (-152.2442, 101.3818) -> (-151.8614, 101.5601) centre (-152.7534, 102.9751) ccw projected
  arc A52 (-153.1756, 101.2399) -> (-152.2442, 101.3818) centre (-153.1548, 104.2313) ccw projected
  arc A53 (-153.5202, 101.714) -> (-153.1756, 101.2399) centre (-148.5, 105) ccw projected
  arc A54 (-153.0974, 102.5559) -> (-153.5202, 101.714) centre (-150.6687, 100.8093) ccw projected
  arc A55 (-152.8095, 102.8649) -> (-153.0974, 102.5559) centre (-151.7394, 101.5794) ccw projected
  arc A56 (-152.6903, 102.9423) -> (-152.8095, 102.8649) centre (-152.4263, 102.4046) ccw projected
  line L14 (-152.6903, 102.9423) -> (-151.8663, 103.3467) projected
  arc A57 (-152.1949, 104.3576) -> (-151.8663, 103.3467) centre (-148.5, 105) ccw projected
  line L15 (-152.1949, 104.3576) -> (-153.0993, 104.2004) projected
  arc A58 (-153.2414, 104.1928) -> (-153.0993, 104.2004) centre (-153.2019, 104.7905) ccw projected
  arc A59 (-153.6559, 104.2736) -> (-153.2414, 104.1928) centre (-153.1313, 105.8619) ccw projected
  arc A60 (-154.4928, 104.7063) -> (-153.6559, 104.2736) centre (-152.7177, 107.1142) ccw projected
  arc A61 (-154.4929, 105.2923) -> (-154.4928, 104.7063) centre (-148.5, 105) ccw projected
  arc A62 (-153.656, 105.725) -> (-154.4929, 105.2923) centre (-152.7177, 102.8844) ccw projected
  arc A63 (-153.2414, 105.8058) -> (-153.656, 105.725) centre (-153.1314, 104.1367) ccw projected
  arc A64 (-153.0995, 105.7982) -> (-153.2414, 105.8058) centre (-153.202, 105.2081) ccw projected
  line L16 (-153.0995, 105.7982) -> (-152.1951, 105.6411) projected
  arc A65 (-151.8668, 106.6521) -> (-152.1951, 105.6411) centre (-148.5, 105) ccw projected
  line L17 (-151.8668, 106.6521) -> (-152.691, 107.0565) projected
  arc A66 (-152.8103, 107.1339) -> (-152.691, 107.0565) centre (-152.4271, 107.5943) ccw projected
  arc A67 (-153.0982, 107.4429) -> (-152.8103, 107.1339) centre (-151.7402, 108.4195) ccw projected
  arc A68 (-153.5209, 108.2848) -> (-153.0982, 107.4429) centre (-150.6695, 109.1895) ccw projected
  arc A69 (-153.1765, 108.759) -> (-153.5209, 108.2848) centre (-148.5, 105) ccw projected
  arc A70 (-152.2451, 108.6171) -> (-153.1765, 108.759) centre (-153.1557, 105.7676) ccw projected
  arc A71 (-151.8623, 108.4388) -> (-152.2451, 108.6171) centre (-152.7543, 107.0239) ccw projected
  arc A72 (-151.7519, 108.3493) -> (-151.8623, 108.4388) centre (-152.1817, 107.9321) ccw projected
  line L18 (-151.7519, 108.3493) -> (-151.1126, 107.6906) projected
  arc A73 (-150.2528, 108.3155) -> (-151.1126, 107.6906) centre (-148.5, 105) ccw projected
  line L19 (-150.2528, 108.3155) -> (-150.6818, 109.1272) projected
  arc A74 (-150.7328, 109.2599) -> (-150.6818, 109.1272) centre (-150.1522, 109.4071) ccw projected
  arc A75 (-150.7841, 109.6791) -> (-150.7328, 109.2599) centre (-149.1115, 109.671) ccw projected
  arc A76 (-150.6312, 110.6087) -> (-150.7841, 109.6791) centre (-147.7926, 109.6645) ccw projected
  arc A77 (-150.0725, 110.7903) -> (-150.6312, 110.6087) centre (-148.5, 105) ccw projected
  arc A78 (-149.402, 110.1264) -> (-150.0725, 110.7903) centre (-151.8157, 108.3591) ccw projected
  arc A79 (-149.1982, 109.7586) -> (-149.402, 110.1264) centre (-150.7515, 109.1382) ccw projected
  arc A80 (-149.1615, 109.6213) -> (-149.1982, 109.7586) centre (-149.7545, 109.5365) ccw projected
  arc A81 (-148.7771, 124.6719) -> (-148.9109, 125.0429) centre (-154.869, 122.6849) ccw projected
  arc A82 (-148.6896, 124.3741) -> (-148.7771, 124.6719) centre (-153.7892, 123.0371) ccw projected
  arc A83 (-148.3104, 124.3741) -> (-148.6896, 124.3741) centre (-148.5, 105) ccw projected
  arc A84 (-148.2229, 124.6719) -> (-148.3104, 124.3741) centre (-143.2108, 123.0371) ccw projected
  arc A85 (-148.0891, 125.0429) -> (-148.2229, 124.6719) centre (-142.131, 122.6849) ccw projected
  arc A86 (-147.8948, 125.4911) -> (-148.0891, 125.0429) centre (-141.0342, 122.2508) ccw projected
  arc A87 (-147.4956, 125.4754) -> (-147.8948, 125.4911) centre (-148.5, 105) ccw projected
  arc A88 (-147.3371, 125.0133) -> (-147.4956, 125.4754) centre (-154.5894, 122.7834) ccw projected
  arc A89 (-147.2329, 124.633) -> (-147.3371, 125.0133) centre (-153.4618, 123.1301) ccw projected
  arc A90 (-147.169, 124.3292) -> (-147.2329, 124.633) centre (-152.3577, 123.3965) ccw projected
  arc A91 (-146.7909, 124.2995) -> (-147.169, 124.3292) centre (-148.5, 105) ccw projected
  arc A92 (-146.6803, 124.5895) -> (-146.7909, 124.2995) centre (-141.8119, 122.5665) ccw projected
  arc A93 (-146.5178, 124.9489) -> (-146.6803, 124.5895) centre (-140.7631, 122.1307) ccw projected
  arc A94 (-146.2889, 125.3804) -> (-146.5178, 124.9489) centre (-139.7037, 121.6119) ccw projected
  arc A95 (-145.8922, 125.3335) -> (-146.2889, 125.3804) centre (-148.5, 105) ccw projected
  arc A96 (-145.7705, 124.8604) -> (-145.8922, 125.3335) centre (-153.1753, 123.2064) ccw projected
  arc A97 (-145.6964, 124.473) -> (-145.7705, 124.8604) centre (-152.0241, 123.4635) ccw projected
  arc A98 (-145.6565, 124.1652) -> (-145.6964, 124.473) centre (-150.9025, 123.6425) ccw projected
  arc A99 (-145.2819, 124.1059) -> (-145.6565, 124.1652) centre (-148.5, 105) ccw projected
  arc A100 (-145.1489, 124.3863) -> (-145.2819, 124.1059) centre (-140.4543, 121.9876) ccw projected
  arc A101 (-144.9587, 124.7318) -> (-145.1489, 124.3863) centre (-139.4429, 121.4708) ccw projected
  arc A102 (-144.6967, 125.1441) -> (-144.9587, 124.7318) centre (-138.4274, 120.8705) ccw projected
  arc A103 (-144.3049, 125.0662) -> (-144.6967, 125.1441) centre (-148.5, 105) ccw projected
  arc A104 (-144.2207, 124.585) -> (-144.3049, 125.0662) centre (-151.7324, 123.517) ccw projected
  arc A105 (-144.1772, 124.193) -> (-144.2207, 124.585) centre (-150.5646, 123.6831) ccw projected
  arc A106 (-144.1616, 123.883) -> (-144.1772, 124.193) centre (-149.4324, 123.7735) ccw projected
  arc A107 (-143.7928, 123.7945) -> (-144.1616, 123.883) centre (-148.5, 105) ccw projected
  arc A108 (-143.6382, 124.0636) -> (-143.7928, 123.7945) centre (-139.1463, 121.304) ccw projected
  arc A109 (-143.4215, 124.3932) -> (-143.6382, 124.0636) centre (-138.1785, 120.7095) ccw projected
  arc A110 (-143.128, 124.7836) -> (-143.4215, 124.3932) centre (-137.2133, 120.0313) ccw projected
  arc A111 (-142.7435, 124.6752) -> (-143.128, 124.7836) centre (-148.5, 105) ccw projected
  arc A112 (-142.6972, 124.1889) -> (-142.7435, 124.6752) centre (-150.2696, 123.7136) ccw projected
  arc A113 (-142.6846, 123.7947) -> (-142.6972, 124.1889) centre (-149.0924, 123.7875) ccw projected
  arc A114 (-142.6934, 123.4844) -> (-142.6846, 123.7947) centre (-147.9566, 123.7888) ccw projected
  arc A115 (-142.3327, 123.3672) -> (-142.6934, 123.4844) centre (-148.5, 105) ccw projected
  arc A116 (-142.1575, 123.6234) -> (-142.3327, 123.3672) centre (-137.8959, 120.5199) ccw projected
  arc A117 (-141.9156, 123.9349) -> (-142.1575, 123.6234) centre (-136.9778, 119.8512) ccw projected
  arc A118 (-141.5923, 124.3011) -> (-141.9156, 123.9349) centre (-136.0688, 119.0994) ccw projected
  arc A119 (-141.2175, 124.1629) -> (-141.5923, 124.3011) centre (-148.5, 105) ccw projected
  arc A120 (-141.2096, 123.6745) -> (-141.2175, 124.1629) centre (-148.7959, 123.7947) ccw projected
  arc A121 (-141.228, 123.2805) -> (-141.2096, 123.6745) centre (-147.6165, 123.776) ccw projected
  arc A122 (-141.2611, 122.9719) -> (-141.228, 123.2805) centre (-146.4841, 123.6882) ccw projected
  arc A123 (-140.9107, 122.8267) -> (-141.2611, 122.9719) centre (-148.5, 105) ccw projected
  arc A124 (-140.7158, 123.0684) -> (-140.9107, 122.8267) centre (-136.7109, 119.64) ccw projected
  arc A125 (-140.4503, 123.36) -> (-140.7158, 123.0684) centre (-135.8481, 118.9014) ccw projected
  arc A126 (-140.0993, 123.6997) -> (-140.4503, 123.36) centre (-135.0009, 118.0806) ccw projected
  arc A127 (-139.7365, 123.5324) -> (-140.0993, 123.6997) centre (-148.5, 105) ccw projected
  arc A128 (-139.7669, 123.0449) -> (-139.7365, 123.5324) centre (-147.3204, 123.76) ccw projected
  arc A129 (-139.8161, 122.6536) -> (-139.7669, 123.0449) centre (-146.1461, 123.6488) ccw projected
  arc A130 (-139.8733, 122.3485) -> (-139.8161, 122.6536) centre (-145.024, 123.4724) ccw projected
  arc A131 (-139.5354, 122.1763) -> (-139.8733, 122.3485) centre (-148.5, 105) ccw projected
  arc A132 (-139.3222, 122.4019) -> (-139.5354, 122.1763) centre (-135.5986, 118.6699) ccw projected
  arc A133 (-139.0346, 122.6718) -> (-139.3222, 122.4019) centre (-134.7964, 117.8659) ccw projected
  arc A134 (-138.658, 122.9829) -> (-139.0346, 122.6718) centre (-134.0162, 116.9812) ccw projected
  arc A135 (-138.3095, 122.7877) -> (-138.658, 122.9829) centre (-148.5, 105) ccw projected
  arc A136 (-138.378, 122.3041) -> (-138.3095, 122.7877) centre (-145.8522, 123.6096) ccw projected
  arc A137 (-138.4578, 121.9178) -> (-138.378, 122.3041) centre (-144.6901, 123.4067) ccw projected
  arc A138 (-138.5388, 121.6182) -> (-138.4578, 121.9178) centre (-143.5854, 123.1428) ccw projected
  arc A139 (-138.2154, 121.42) -> (-138.5388, 121.6182) centre (-148.5, 105) ccw projected
  arc A140 (-137.9852, 121.6282) -> (-138.2154, 121.42) centre (-134.5659, 117.6156) ccw projected
  arc A141 (-137.6773, 121.8747) -> (-137.9852, 121.6282) centre (-133.8292, 116.7511) ccw projected
  arc A142 (-137.2774, 122.1553) -> (-137.6773, 121.8747) centre (-133.1208, 115.8078) ccw projected
  arc A143 (-136.9453, 121.9334) -> (-137.2774, 122.1553) centre (-148.5, 105) ccw projected
  arc A144 (-137.0515, 121.4566) -> (-136.9453, 121.9334) centre (-144.4002, 123.3445) ccw projected
  arc A145 (-137.1614, 121.0778) -> (-137.0515, 121.4566) centre (-143.2577, 123.051) ccw projected
  arc A146 (-137.2656, 120.7854) -> (-137.1614, 121.0778) centre (-142.1771, 122.7012) ccw projected
  arc A147 (-136.9588, 120.5625) -> (-137.2656, 120.7854) centre (-148.5, 105) ccw projected
  arc A148 (-136.7129, 120.752) -> (-136.9588, 120.5625) centre (-133.619, 116.4834) ccw projected
  arc A149 (-136.3866, 120.9735) -> (-136.7129, 120.752) centre (-132.9524, 115.5638) ccw projected
  arc A150 (-135.966, 121.2219) -> (-136.3866, 120.9735) centre (-132.3202, 114.5679) ccw projected
  arc A151 (-135.6523, 120.9746) -> (-135.966, 121.2219) centre (-148.5, 105) ccw projected
  arc A152 (-135.7957, 120.5076) -> (-135.6523, 120.9746) centre (-142.9736, 122.9663) ccw projected
  arc A153 (-135.9349, 120.1386) -> (-135.7957, 120.5076) centre (-141.8576, 122.5841) ccw projected
  arc A154 (-136.0617, 119.8553) -> (-135.9349, 120.1386) centre (-140.8078, 122.1506) ccw projected
  arc A155 (-135.7734, 119.609) -> (-136.0617, 119.8553) centre (-148.5, 105) ccw projected
  arc A156 (-135.5134, 119.7786) -> (-135.7734, 119.609) centre (-132.7639, 115.2805) ccw projected
  arc A157 (-135.1707, 119.9739) -> (-135.5134, 119.7786) centre (-132.1715, 114.3114) ccw projected
  arc A158 (-134.7319, 120.1885) -> (-135.1707, 119.9739) centre (-131.6194, 113.2689) ccw projected
  arc A159 (-134.4386, 119.9173) -> (-134.7319, 120.1885) centre (-148.5, 105) ccw projected
  arc A160 (-134.6181, 119.463) -> (-134.4386, 119.9173) centre (-141.581, 122.4773) ccw projected
  arc A161 (-134.7859, 119.1061) -> (-134.6181, 119.463) centre (-140.4985, 122.0087) ccw projected
  arc A162 (-134.9345, 118.8336) -> (-134.7859, 119.1061) centre (-139.4859, 121.4942) ccw projected
  arc A163 (-134.6664, 118.5655) -> (-134.9345, 118.8336) centre (-148.5, 105) ccw projected
  arc A164 (-134.3939, 118.7141) -> (-134.6664, 118.5655) centre (-132.0058, 114.0141) ccw projected
  arc A165 (-134.037, 118.8819) -> (-134.3939, 118.7141) centre (-131.4913, 113.0015) ccw projected
  arc A166 (-133.5827, 119.0614) -> (-134.037, 118.8819) centre (-131.0227, 111.919) ccw projected
  arc A167 (-133.3115, 118.7681) -> (-133.5827, 119.0614) centre (-148.5, 105) ccw projected
  arc A168 (-133.5261, 118.3293) -> (-133.3115, 118.7681) centre (-140.2311, 121.8806) ccw projected
  arc A169 (-133.7214, 117.9866) -> (-133.5261, 118.3293) centre (-139.1886, 121.3285) ccw projected
  arc A170 (-133.891, 117.7266) -> (-133.7214, 117.9866) centre (-138.2195, 120.7361) ccw projected
  arc A171 (-133.6447, 117.4383) -> (-133.891, 117.7266) centre (-148.5, 105) ccw projected
  arc A172 (-133.3614, 117.5651) -> (-133.6447, 117.4383) centre (-131.3494, 112.6922) ccw projected
  arc A173 (-132.9924, 117.7043) -> (-133.3614, 117.5651) centre (-130.9159, 111.6424) ccw projected
  arc A174 (-132.5254, 117.8477) -> (-132.9924, 117.7043) centre (-130.5337, 110.5264) ccw projected
  arc A175 (-132.2781, 117.534) -> (-132.5254, 117.8477) centre (-148.5, 105) ccw projected
  arc A176 (-132.5265, 117.1134) -> (-132.2781, 117.534) centre (-138.9321, 121.1798) ccw projected
  arc A177 (-132.748, 116.7871) -> (-132.5265, 117.1134) centre (-137.9362, 120.5476) ccw projected
  arc A178 (-132.9375, 116.5412) -> (-132.748, 116.7871) centre (-137.0166, 119.881) ccw projected
  arc A179 (-132.7146, 116.2344) -> (-132.9375, 116.5412) centre (-148.5, 105) ccw projected
  arc A180 (-132.4222, 116.3386) -> (-132.7146, 116.2344) centre (-130.7988, 111.3229) ccw projected
  arc A181 (-132.0434, 116.4485) -> (-132.4222, 116.3386) centre (-130.449, 110.2423) ccw projected
  arc A182 (-131.5666, 116.5547) -> (-132.0434, 116.4485) centre (-130.1555, 109.0998) ccw projected
  arc A183 (-131.3447, 116.2226) -> (-131.5666, 116.5547) centre (-148.5, 105) ccw projected
  arc A184 (-131.6253, 115.8227) -> (-131.3447, 116.2226) centre (-137.6922, 120.3792) ccw projected
  arc A185 (-131.8718, 115.5148) -> (-131.6253, 115.8227) centre (-136.7489, 119.6708) ccw projected
  arc A186 (-132.08, 115.2846) -> (-131.8718, 115.5148) centre (-135.8844, 118.9341) ccw projected
  arc A187 (-131.8818, 114.9612) -> (-132.08, 115.2846) centre (-148.5, 105) ccw projected
  arc A188 (-131.5822, 115.0422) -> (-131.8818, 114.9612) centre (-130.3572, 109.9146) ccw projected
  arc A189 (-131.1959, 115.122) -> (-131.5822, 115.0422) centre (-130.0933, 108.8099) ccw projected
  arc A190 (-130.7123, 115.1905) -> (-131.1959, 115.122) centre (-129.8904, 107.6478) ccw projected
  arc A191 (-130.5171, 114.842) -> (-130.7123, 115.1905) centre (-148.5, 105) ccw projected
  arc A192 (-130.8282, 114.4654) -> (-130.5171, 114.842) centre (-136.5188, 119.4838) ccw projected
  arc A193 (-131.0981, 114.1778) -> (-130.8282, 114.4654) centre (-135.6341, 118.7036) ccw projected
  arc A194 (-131.3237, 113.9646) -> (-131.0981, 114.1778) centre (-134.8301, 117.9014) ccw projected
  arc A195 (-131.1515, 113.6267) -> (-131.3237, 113.9646) centre (-148.5, 105) ccw projected
  arc A196 (-130.8464, 113.6839) -> (-131.1515, 113.6267) centre (-130.0276, 108.476) ccw projected
  arc A197 (-130.4551, 113.7331) -> (-130.8464, 113.6839) centre (-129.8512, 107.3539) ccw projected
  arc A198 (-129.9676, 113.7635) -> (-130.4551, 113.7331) centre (-129.74, 106.1796) ccw projected
  arc A199 (-129.8003, 113.4007) -> (-129.9676, 113.7635) centre (-148.5, 105) ccw projected
  arc A200 (-130.14, 113.0497) -> (-129.8003, 113.4007) centre (-135.4194, 118.4991) ccw projected
  arc A201 (-130.4316, 112.7842) -> (-130.14, 113.0497) centre (-134.5986, 117.6519) ccw projected
  arc A202 (-130.6733, 112.5893) -> (-130.4316, 112.7842) centre (-133.86, 116.7891) ccw projected
  arc A203 (-130.5281, 112.2389) -> (-130.6733, 112.5893) centre (-148.5, 105) ccw projected
  arc A204 (-130.2195, 112.272) -> (-130.5281, 112.2389) centre (-129.8118, 107.0159) ccw projected
  arc A205 (-129.8255, 112.2904) -> (-130.2195, 112.272) centre (-129.724, 105.8835) ccw projected
  arc A206 (-129.3371, 112.2825) -> (-129.8255, 112.2904) centre (-129.7053, 104.7041) ccw projected
  arc A207 (-129.1989, 111.9077) -> (-129.3371, 112.2825) centre (-148.5, 105) ccw projected
  arc A208 (-129.5651, 111.5844) -> (-129.1989, 111.9077) centre (-134.4006, 117.4312) ccw projected
  arc A209 (-129.8766, 111.3425) -> (-129.5651, 111.5844) centre (-133.6488, 116.5222) ccw projected
  arc A210 (-130.1328, 111.1673) -> (-129.8766, 111.3425) centre (-132.9801, 115.6041) ccw projected
  arc A211 (-130.0156, 110.8066) -> (-130.1328, 111.1673) centre (-148.5, 105) ccw projected
  arc A212 (-129.7053, 110.8154) -> (-130.0156, 110.8066) centre (-129.7112, 105.5434) ccw projected
  arc A213 (-129.3111, 110.8028) -> (-129.7053, 110.8154) centre (-129.7125, 104.4076) ccw projected
  arc A214 (-128.8248, 110.7565) -> (-129.3111, 110.8028) centre (-129.7864, 103.2304) ccw projected
  arc A215 (-128.7164, 110.372) -> (-128.8248, 110.7565) centre (-148.5, 105) ccw projected
  arc A216 (-129.1068, 110.0785) -> (-128.7164, 110.372) centre (-133.4687, 116.2867) ccw projected
  arc A217 (-129.4364, 109.8618) -> (-129.1068, 110.0785) centre (-132.7905, 115.3215) ccw projected
  arc A218 (-129.7055, 109.7072) -> (-129.4364, 109.8618) centre (-132.196, 114.3537) ccw projected
  arc A219 (-129.617, 109.3384) -> (-129.7055, 109.7072) centre (-148.5, 105) ccw projected
  arc A220 (-129.307, 109.3228) -> (-129.617, 109.3384) centre (-129.7265, 104.0676) ccw projected
  arc A221 (-128.915, 109.2793) -> (-129.307, 109.3228) centre (-129.8169, 102.9354) ccw projected
  arc A222 (-128.4338, 109.1951) -> (-128.915, 109.2793) centre (-129.983, 101.7676) ccw projected
  arc A223 (-128.3559, 108.8033) -> (-128.4338, 109.1951) centre (-148.5, 105) ccw projected
  arc A224 (-128.7682, 108.5413) -> (-128.3559, 108.8033) centre (-132.6295, 115.0726) ccw projected
  arc A225 (-129.1137, 108.3511) -> (-128.7682, 108.5413) centre (-132.0292, 114.0571) ccw projected
  arc A226 (-129.3941, 108.2181) -> (-129.1137, 108.3511) centre (-131.5124, 113.0457) ccw projected
  arc A227 (-129.3348, 107.8435) -> (-129.3941, 108.2181) centre (-148.5, 105) ccw projected
  arc A228 (-129.027, 107.8036) -> (-129.3348, 107.8435) centre (-129.8575, 102.5975) ccw projected